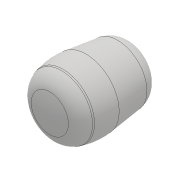
# Autodesk Inventor part: insideFront
Saved by Autodesk Inventor 2017 (Build 210142000, 142)
## iProperties
Created: 2018-06-30
Part Number: insideFront
Material: Generic
Document SubType Name: Modeling
Designer: mfans
Density: 1 g/cm^3
Appearance: Default
Author: mfans
Autodesk Inventor part; units mm, degrees
ref_plane "YZ Plane" through (0, 0, 0) normal (1, 0, 0) x (0, 1, 0)
ref_plane "XZ Plane" through (0, 0, 0) normal (0, 1, 0) x (-1, 0, 0)
ref_plane "XY Plane" through (0, 0, 0) normal (0, 0, 1) x (1, 0, 0)
sketch "Sketch1" plane through (0, 0, 0) normal (0, 0, 1) x (1, 0, 0)
  line L0 (0, 0) -> (40, 0)
  arc A0 (0, -9.4427) -> (40, 0) centre (0, 80) ccw
  line L1 (40, 0) -> (30, 80)
  line L2 (30, 80) -> (0, 80)
  line L3 (0, 80) -> (0, -9.4427)
  dimension "d0" = 40
  dimension "d1" = 80
  dimension "d2" = 30
  constraints: 8 end point, 2 horizontal, 2 point on circle, 1 centre point, 1 perpendicular
  measures "d0" distance of L0.start L0.end
  measures "d1" distance of L0.start L2.end
  measures "d2" distance of L1.end L2.end
revolve "Revolution1" add sketch "Sketch1" angle 360 about axis through (0, 80, 0) along (0, -1, 0)
fillet "Fillet1" radius 20 1 edges at (-30, 80, 0)
chamfer "Chamfer1" distance 10 distance2 20 1 edges at (-40, 0, 0) measured on face at (-39.5522, -0.2224, 0)
fillet "Fillet2" radius 20 1 edges at (-30.8197, -3.9651, 0)
fillet "Fillet3" radius 60 1 edges at (-37.5193, 19.8456, 0)
thicken "Thicken1" operation add thickness 4 both sides no extend neighbours yes toward (0.424649, -0.203286, -0.8822404) faces at (-13.8468, 64.0657, 28.7677) (-19.2562, 38.6738, 29.425) (19.6833, 27.9174, -30.5928) (23.3294, 7.1826, -24.6734) (33.0587, 5.0901, 3.9555) (12.8555, -8.4033, -4.4259) (-4.9872, 80, -0.9847)
body "Solid1"
